Autodesk Inventor part; units mm, degrees
(part 2 of 2)
  spline S263 degree 2 poles (-39.5849, -51.31) (-39.1944, -51.6609) (-38.794, -52.3233) (-38.794, -52.7089) knots 0 0 0 1 2 2 2
  spline S264 degree 2 poles (-38.794, -52.7089) (-38.794, -53.0055) (-38.9769, -53.49) (-39.1845, -53.6679) knots 0 0 0 1 2 2 2
  spline S265 degree 2 poles (-39.1845, -53.6679) (-39.3921, -53.8508) (-40.015, -54.0535) (-40.4846, -54.0535) knots 0 0 0 1 2 2 2
  line L187 (-40.4846, -54.0535) -> (-43.5, -54.0535)
  line L188 (-43.5, -54.0535) -> (-43.5, -53.2823)
  line L189 (-43.5, -60.3265) -> (-40.8504, -60.3265)
  spline S266 degree 2 poles (-40.8504, -60.3265) (-40.534, -60.3265) (-39.9952, -60.2771) (-39.8469, -60.198) knots 0 0 0 1 2 2 2
  spline S267 degree 2 poles (-39.8469, -60.198) (-39.6838, -60.1189) (-39.5256, -59.8173) (-39.5256, -59.5553) knots 0 0 0 1 2 2 2
  spline S268 degree 2 poles (-39.5256, -59.5553) (-39.5256, -59.3181) (-39.8173, -58.7743) (-40.0941, -58.4876) knots 0 0 0 1 2 2 2
  spline S269 degree 2 poles (-40.0941, -58.4876) (-40.1633, -58.4925) (-40.3561, -58.5024) (-40.4846, -58.5024) knots 0 0 0 1 2 2 2
  line L190 (-40.4846, -58.5024) -> (-43.5, -58.5024)
  line L191 (-43.5, -58.5024) -> (-43.5, -57.7313)
  line L192 (-43.5, -57.7313) -> (-40.8504, -57.7313)
  spline S270 degree 2 poles (-40.8504, -57.7313) (-40.534, -57.7313) (-39.9952, -57.6818) (-39.8469, -57.6028) knots 0 0 0 1 2 2 2
  spline S271 degree 2 poles (-39.8469, -57.6028) (-39.6838, -57.5237) (-39.5256, -57.2221) (-39.5256, -56.9601) knots 0 0 0 1 2 2 2
  spline S272 degree 2 poles (-39.5256, -56.9601) (-39.5256, -56.713) (-39.837, -56.1643) (-40.0793, -55.9072) knots 0 0 0 1 2 2 2
  line L193 (-40.0793, -55.9072) -> (-43.5, -55.9072)
  line L194 (-43.5, -55.9072) -> (-43.5, -55.1361)
  line L195 (-43.5, -55.1361) -> (-38.9225, -55.1361)
  line L196 (-38.9225, -55.1361) -> (-38.9225, -55.9072)
  line L197 (-38.9225, -55.9072) -> (-39.4267, -55.9072)
  spline S273 degree 2 poles (-39.4267, -55.9072) (-39.1252, -56.2088) (-38.794, -56.8019) (-38.794, -57.1579) knots 0 0 0 1 2 2 2
  spline S274 degree 2 poles (-38.794, -57.1579) (-38.794, -57.5632) (-39.1647, -58.191) (-39.5849, -58.3541) knots 0 0 0 1 2 2 2
  spline S275 degree 2 poles (-39.5849, -58.3541) (-39.1944, -58.7051) (-38.794, -59.3675) (-38.794, -59.7531) knots 0 0 0 1 2 2 2
  spline S276 degree 2 poles (-38.794, -59.7531) (-38.794, -60.0497) (-38.9769, -60.5341) (-39.1845, -60.7121) knots 0 0 0 1 2 2 2
  spline S277 degree 2 poles (-39.1845, -60.7121) (-39.3921, -60.895) (-40.015, -61.0976) (-40.4846, -61.0976) knots 0 0 0 1 2 2 2
  line L198 (-40.4846, -61.0976) -> (-43.5, -61.0976)
  line L199 (-43.5, -61.0976) -> (-43.5, -60.3265)
  spline S278 degree 2 poles (-53.6384, -40.6671) (-53.6384, -40.2123) (-53.3665, -39.4659) (-53.1144, -39.2039) knots 0 0 0 1 2 2 2
  spline S279 degree 2 poles (-53.1144, -39.2039) (-52.8673, -38.9468) (-52.195, -38.6799) (-51.8143, -38.6799) knots 0 0 0 1 2 2 2
  spline S280 degree 2 poles (-51.8143, -38.6799) (-51.32, -38.6799) (-50.4895, -39.2088) (-50.2424, -39.713) knots 0 0 0 1 2 2 2
  line L200 (-50.2424, -39.713) -> (-50.2177, -39.713)
  spline S281 degree 2 poles (-50.2177, -39.713) (-49.9557, -39.2632) (-49.3328, -38.8282) (-48.8682, -38.8282) knots 0 0 0 1 2 2 2
  spline S282 degree 2 poles (-48.8682, -38.8282) (-48.181, -38.8282) (-47.2616, -39.8663) (-47.2616, -40.6671) knots 0 0 0 1 2 2 2
  spline S283 degree 2 poles (-47.2616, -40.6671) (-47.2616, -41.4976) (-48.1316, -42.5011) (-48.8138, -42.5011) knots 0 0 0 1 2 2 2
  spline S284 degree 2 poles (-48.8138, -42.5011) (-49.2241, -42.5011) (-50.0249, -42.0216) (-50.2523, -41.5717) knots 0 0 0 1 2 2 2
  line L201 (-50.2523, -41.5717) -> (-50.277, -41.5717)
  spline S285 degree 2 poles (-50.277, -41.5717) (-50.5241, -42.1056) (-51.236, -42.6543) (-51.7995, -42.6543) knots 0 0 0 1 2 2 2
  spline S286 degree 2 poles (-51.7995, -42.6543) (-52.5806, -42.6543) (-53.6384, -41.5173) (-53.6384, -40.6671) knots 0 0 0 1 2 2 2
  spline S287 degree 2 poles (-51.8786, -41.8139) (-51.5029, -41.8139) (-51.058, -41.5173) (-50.8306, -41.0972) knots 0 0 0 1 2 2 2
  spline S288 degree 2 poles (-50.8306, -41.0972) (-50.7515, -40.9588) (-50.5686, -40.4941) (-50.45, -40.2024) knots 0 0 0 1 2 2 2
  spline S289 degree 2 poles (-50.45, -40.2024) (-50.6724, -39.8663) (-51.3348, -39.5054) (-51.755, -39.5054) knots 0 0 0 1 2 2 2
  spline S290 degree 2 poles (-51.755, -39.5054) (-52.3087, -39.5054) (-53.0304, -40.1728) (-53.0304, -40.677) knots 0 0 0 1 2 2 2
  spline S291 degree 2 poles (-53.0304, -40.677) (-53.0304, -41.1911) (-52.4125, -41.8139) (-51.8786, -41.8139) knots 0 0 0 1 2 2 2
  spline S292 degree 2 poles (-48.8237, -41.7002) (-48.4134, -41.7002) (-47.8647, -41.1515) (-47.8647, -40.6622) knots 0 0 0 1 2 2 2
  spline S293 degree 2 poles (-47.8647, -40.6622) (-47.8647, -40.2173) (-48.3541, -39.6488) (-48.7742, -39.6488) knots 0 0 0 1 2 2 2
  spline S294 degree 2 poles (-48.7742, -39.6488) (-49.0758, -39.6488) (-49.4959, -39.9404) (-49.664, -40.2321) knots 0 0 0 1 2 2 2
  spline S295 degree 2 poles (-49.664, -40.2321) (-49.7332, -40.3557) (-49.9754, -40.8797) (-50.0447, -41.0922) knots 0 0 0 1 2 2 2
  spline S296 degree 2 poles (-50.0447, -41.0922) (-49.7728, -41.4481) (-49.1944, -41.7002) (-48.8237, -41.7002) knots 0 0 0 1 2 2 2
  spline S297 degree 2 poles (-50.45, -47.1972) (-52.0912, -47.1972) (-53.6285, -46.2431) (-53.6285, -45.2495) knots 0 0 0 1 2 2 2
  spline S298 degree 2 poles (-53.6285, -45.2495) (-53.6285, -44.2411) (-52.0615, -43.2969) (-50.4549, -43.2969) knots 0 0 0 1 2 2 2
  spline S299 degree 2 poles (-50.4549, -43.2969) (-48.8039, -43.2969) (-47.2764, -44.251) (-47.2764, -45.2495) knots 0 0 0 1 2 2 2
  spline S300 degree 2 poles (-47.2764, -45.2495) (-47.2764, -46.253) (-48.8583, -47.1972) (-50.45, -47.1972) knots 0 0 0 1 2 2 2
  spline S301 degree 2 poles (-52.3087, -46.1492) (-52.0071, -46.2678) (-51.0778, -46.3667) (-50.45, -46.3667) knots 0 0 0 1 2 2 2
  spline S302 degree 2 poles (-50.45, -46.3667) (-49.8222, -46.3667) (-48.8978, -46.2678) (-48.5864, -46.1442) knots 0 0 0 1 2 2 2
  spline S303 degree 2 poles (-48.5864, -46.1442) (-48.275, -46.0207) (-47.9536, -45.5906) (-47.9536, -45.2495) knots 0 0 0 1 2 2 2
  spline S304 degree 2 poles (-47.9536, -45.2495) (-47.9536, -44.9084) (-48.275, -44.4685) (-48.5963, -44.34) knots 0 0 0 1 2 2 2
  spline S305 degree 2 poles (-48.5963, -44.34) (-48.9077, -44.2164) (-49.8568, -44.1274) (-50.4549, -44.1274) knots 0 0 0 1 2 2 2
  spline S306 degree 2 poles (-50.4549, -44.1274) (-51.0976, -44.1274) (-51.9577, -44.2065) (-52.2938, -44.335) knots 0 0 0 1 2 2 2
  spline S307 degree 2 poles (-52.2938, -44.335) (-52.6102, -44.4536) (-52.9513, -44.8936) (-52.9513, -45.2495) knots 0 0 0 1 2 2 2
  spline S308 degree 2 poles (-52.9513, -45.2495) (-52.9513, -45.5857) (-52.63, -46.0256) (-52.3087, -46.1492) knots 0 0 0 1 2 2 2
  line L202 (-53.5, -53.2823) -> (-50.8504, -53.2823)
  spline S309 degree 2 poles (-50.8504, -53.2823) (-50.534, -53.2823) (-49.9952, -53.2329) (-49.8469, -53.1538) knots 0 0 0 1 2 2 2
  spline S310 degree 2 poles (-49.8469, -53.1538) (-49.6838, -53.0747) (-49.5256, -52.7732) (-49.5256, -52.5112) knots 0 0 0 1 2 2 2
  spline S311 degree 2 poles (-49.5256, -52.5112) (-49.5256, -52.2739) (-49.8173, -51.7301) (-50.0941, -51.4434) knots 0 0 0 1 2 2 2
  spline S312 degree 2 poles (-50.0941, -51.4434) (-50.1633, -51.4484) (-50.3561, -51.4583) (-50.4846, -51.4583) knots 0 0 0 1 2 2 2
  line L203 (-50.4846, -51.4583) -> (-53.5, -51.4583)
  line L204 (-53.5, -51.4583) -> (-53.5, -50.6871)
  line L205 (-53.5, -50.6871) -> (-50.8504, -50.6871)
  spline S313 degree 2 poles (-50.8504, -50.6871) (-50.534, -50.6871) (-49.9952, -50.6377) (-49.8469, -50.5586) knots 0 0 0 1 2 2 2
  spline S314 degree 2 poles (-49.8469, -50.5586) (-49.6838, -50.4795) (-49.5256, -50.178) (-49.5256, -49.916) knots 0 0 0 1 2 2 2
  spline S315 degree 2 poles (-49.5256, -49.916) (-49.5256, -49.6688) (-49.837, -49.1201) (-50.0793, -48.863) knots 0 0 0 1 2 2 2
  line L206 (-50.0793, -48.863) -> (-53.5, -48.863)
  line L207 (-53.5, -48.863) -> (-53.5, -48.0919)
  line L208 (-53.5, -48.0919) -> (-48.9225, -48.0919)
  line L209 (-48.9225, -48.0919) -> (-48.9225, -48.863)
  line L210 (-48.9225, -48.863) -> (-49.4267, -48.863)
  spline S316 degree 2 poles (-49.4267, -48.863) (-49.1252, -49.1646) (-48.794, -49.7578) (-48.794, -50.1137) knots 0 0 0 1 2 2 2
  spline S317 degree 2 poles (-48.794, -50.1137) (-48.794, -50.519) (-49.1647, -51.1468) (-49.5849, -51.31) knots 0 0 0 1 2 2 2
  spline S318 degree 2 poles (-49.5849, -51.31) (-49.1944, -51.6609) (-48.794, -52.3233) (-48.794, -52.7089) knots 0 0 0 1 2 2 2
  spline S319 degree 2 poles (-48.794, -52.7089) (-48.794, -53.0055) (-48.9769, -53.49) (-49.1845, -53.6679) knots 0 0 0 1 2 2 2
  spline S320 degree 2 poles (-49.1845, -53.6679) (-49.3921, -53.8508) (-50.015, -54.0535) (-50.4846, -54.0535) knots 0 0 0 1 2 2 2
  line L211 (-50.4846, -54.0535) -> (-53.5, -54.0535)
  line L212 (-53.5, -54.0535) -> (-53.5, -53.2823)
  line L213 (-53.5, -60.3265) -> (-50.8504, -60.3265)
  spline S321 degree 2 poles (-50.8504, -60.3265) (-50.534, -60.3265) (-49.9952, -60.2771) (-49.8469, -60.198) knots 0 0 0 1 2 2 2
  spline S322 degree 2 poles (-49.8469, -60.198) (-49.6838, -60.1189) (-49.5256, -59.8173) (-49.5256, -59.5553) knots 0 0 0 1 2 2 2
  spline S323 degree 2 poles (-49.5256, -59.5553) (-49.5256, -59.3181) (-49.8173, -58.7743) (-50.0941, -58.4876) knots 0 0 0 1 2 2 2
  spline S324 degree 2 poles (-50.0941, -58.4876) (-50.1633, -58.4925) (-50.3561, -58.5024) (-50.4846, -58.5024) knots 0 0 0 1 2 2 2
  line L214 (-50.4846, -58.5024) -> (-53.5, -58.5024)
  line L215 (-53.5, -58.5024) -> (-53.5, -57.7313)
  line L216 (-53.5, -57.7313) -> (-50.8504, -57.7313)
  spline S325 degree 2 poles (-50.8504, -57.7313) (-50.534, -57.7313) (-49.9952, -57.6818) (-49.8469, -57.6028) knots 0 0 0 1 2 2 2
  spline S326 degree 2 poles (-49.8469, -57.6028) (-49.6838, -57.5237) (-49.5256, -57.2221) (-49.5256, -56.9601) knots 0 0 0 1 2 2 2
  spline S327 degree 2 poles (-49.5256, -56.9601) (-49.5256, -56.713) (-49.837, -56.1643) (-50.0793, -55.9072) knots 0 0 0 1 2 2 2
  line L217 (-50.0793, -55.9072) -> (-53.5, -55.9072)
  line L218 (-53.5, -55.9072) -> (-53.5, -55.1361)
  line L219 (-53.5, -55.1361) -> (-48.9225, -55.1361)
  line L220 (-48.9225, -55.1361) -> (-48.9225, -55.9072)
  line L221 (-48.9225, -55.9072) -> (-49.4267, -55.9072)
  spline S328 degree 2 poles (-49.4267, -55.9072) (-49.1252, -56.2088) (-48.794, -56.8019) (-48.794, -57.1579) knots 0 0 0 1 2 2 2
  spline S329 degree 2 poles (-48.794, -57.1579) (-48.794, -57.5632) (-49.1647, -58.191) (-49.5849, -58.3541) knots 0 0 0 1 2 2 2
  spline S330 degree 2 poles (-49.5849, -58.3541) (-49.1944, -58.7051) (-48.794, -59.3675) (-48.794, -59.7531) knots 0 0 0 1 2 2 2
  spline S331 degree 2 poles (-48.794, -59.7531) (-48.794, -60.0497) (-48.9769, -60.5341) (-49.1845, -60.7121) knots 0 0 0 1 2 2 2
  spline S332 degree 2 poles (-49.1845, -60.7121) (-49.3921, -60.895) (-50.015, -61.0976) (-50.4846, -61.0976) knots 0 0 0 1 2 2 2
  line L222 (-50.4846, -61.0976) -> (-53.5, -61.0976)
  line L223 (-53.5, -61.0976) -> (-53.5, -60.3265)
  spline S333 degree 2 poles (-59.3823, -38.6552) (-58.9126, -38.6552) (-58.1316, -38.9617) (-57.8498, -39.2286) knots 0 0 0 1 2 2 2
  spline S334 degree 2 poles (-57.8498, -39.2286) (-57.578, -39.4807) (-57.2764, -40.2173) (-57.2764, -40.5929) knots 0 0 0 1 2 2 2
  spline S335 degree 2 poles (-57.2764, -40.5929) (-57.2764, -41.0131) (-57.5582, -41.6953) (-57.8251, -41.9474) knots 0 0 0 1 2 2 2
  spline S336 degree 2 poles (-57.8251, -41.9474) (-58.1613, -42.2638) (-59.2488, -42.6098) (-60.0842, -42.6098) knots 0 0 0 1 2 2 2
  spline S337 degree 2 poles (-60.0842, -42.6098) (-60.8405, -42.6098) (-62.195, -42.2687) (-62.6448, -41.9375) knots 0 0 0 1 2 2 2
  spline S338 degree 2 poles (-62.6448, -41.9375) (-63.1194, -41.5865) (-63.6186, -40.5979) (-63.6186, -39.8762) knots 0 0 0 1 2 2 2
  spline S339 degree 2 poles (-63.6186, -39.8762) (-63.6186, -39.713) (-63.584, -39.3423) (-63.5346, -39.1841) knots 0 0 0 1 2 2 2
  line L224 (-63.5346, -39.1841) -> (-62.7486, -39.1841)
  line L225 (-62.7486, -39.1841) -> (-62.7486, -39.2237)
  spline S340 degree 2 poles (-62.7486, -39.2237) (-62.8079, -39.3275) (-62.9118, -39.7625) (-62.9118, -39.9849) knots 0 0 0 1 2 2 2
  spline S341 degree 2 poles (-62.9118, -39.9849) (-62.9118, -40.7857) (-61.8539, -41.7002) (-60.8751, -41.7645) knots 0 0 0 1 2 2 2
  spline S342 degree 2 poles (-60.8751, -41.7645) (-61.0976, -41.4382) (-61.3002, -40.8451) (-61.3002, -40.4941) knots 0 0 0 1 2 2 2
  spline S343 degree 2 poles (-61.3002, -40.4941) (-61.3002, -40.1579) (-61.1519, -39.5994) (-60.9394, -39.3176) knots 0 0 0 1 2 2 2
  spline S344 degree 2 poles (-60.9394, -39.3176) (-60.6873, -38.9913) (-59.9211, -38.6552) (-59.3823, -38.6552) knots 0 0 0 1 2 2 2
  spline S345 degree 2 poles (-59.9013, -41.7843) (-59.2834, -41.7843) (-58.5023, -41.5569) (-58.2898, -41.3542) knots 0 0 0 1 2 2 2
  spline S346 degree 2 poles (-58.2898, -41.3542) (-58.0921, -41.1763) (-57.9438, -40.8055) (-57.9438, -40.588) knots 0 0 0 1 2 2 2
  spline S347 degree 2 poles (-57.9438, -40.588) (-57.9438, -40.0838) (-58.6655, -39.4857) (-59.3476, -39.4857) knots 0 0 0 1 2 2 2
  spline S348 degree 2 poles (-59.3476, -39.4857) (-59.7332, -39.4857) (-60.2325, -39.6834) (-60.4105, -39.9009) knots 0 0 0 1 2 2 2
  spline S349 degree 2 poles (-60.4105, -39.9009) (-60.539, -40.0591) (-60.623, -40.4496) (-60.623, -40.677) knots 0 0 0 1 2 2 2
  spline S350 degree 2 poles (-60.623, -40.677) (-60.623, -40.939) (-60.4401, -41.5421) (-60.2869, -41.7694) knots 0 0 0 1 2 2 2
  spline S351 degree 2 poles (-60.2869, -41.7694) (-60.2276, -41.7744) (-60.0249, -41.7843) (-59.9013, -41.7843) knots 0 0 0 1 2 2 2
  spline S352 degree 2 poles (-60.45, -47.1972) (-62.0912, -47.1972) (-63.6285, -46.2431) (-63.6285, -45.2495) knots 0 0 0 1 2 2 2
  spline S353 degree 2 poles (-63.6285, -45.2495) (-63.6285, -44.2411) (-62.0615, -43.2969) (-60.4549, -43.2969) knots 0 0 0 1 2 2 2
  spline S354 degree 2 poles (-60.4549, -43.2969) (-58.8039, -43.2969) (-57.2764, -44.251) (-57.2764, -45.2495) knots 0 0 0 1 2 2 2
  spline S355 degree 2 poles (-57.2764, -45.2495) (-57.2764, -46.253) (-58.8583, -47.1972) (-60.45, -47.1972) knots 0 0 0 1 2 2 2
  spline S356 degree 2 poles (-62.3087, -46.1492) (-62.0071, -46.2678) (-61.0778, -46.3667) (-60.45, -46.3667) knots 0 0 0 1 2 2 2
  spline S357 degree 2 poles (-60.45, -46.3667) (-59.8222, -46.3667) (-58.8978, -46.2678) (-58.5864, -46.1442) knots 0 0 0 1 2 2 2
  spline S358 degree 2 poles (-58.5864, -46.1442) (-58.275, -46.0207) (-57.9536, -45.5906) (-57.9536, -45.2495) knots 0 0 0 1 2 2 2
  spline S359 degree 2 poles (-57.9536, -45.2495) (-57.9536, -44.9084) (-58.275, -44.4685) (-58.5963, -44.34) knots 0 0 0 1 2 2 2
  spline S360 degree 2 poles (-58.5963, -44.34) (-58.9077, -44.2164) (-59.8568, -44.1274) (-60.4549, -44.1274) knots 0 0 0 1 2 2 2
  spline S361 degree 2 poles (-60.4549, -44.1274) (-61.0976, -44.1274) (-61.9577, -44.2065) (-62.2938, -44.335) knots 0 0 0 1 2 2 2
  spline S362 degree 2 poles (-62.2938, -44.335) (-62.6102, -44.4536) (-62.9513, -44.8936) (-62.9513, -45.2495) knots 0 0 0 1 2 2 2
  spline S363 degree 2 poles (-62.9513, -45.2495) (-62.9513, -45.5857) (-62.63, -46.0256) (-62.3087, -46.1492) knots 0 0 0 1 2 2 2
  line L226 (-63.5, -53.2823) -> (-60.8504, -53.2823)
  spline S364 degree 2 poles (-60.8504, -53.2823) (-60.534, -53.2823) (-59.9952, -53.2329) (-59.8469, -53.1538) knots 0 0 0 1 2 2 2
  spline S365 degree 2 poles (-59.8469, -53.1538) (-59.6838, -53.0747) (-59.5256, -52.7732) (-59.5256, -52.5112) knots 0 0 0 1 2 2 2
  spline S366 degree 2 poles (-59.5256, -52.5112) (-59.5256, -52.2739) (-59.8173, -51.7301) (-60.0941, -51.4434) knots 0 0 0 1 2 2 2
  spline S367 degree 2 poles (-60.0941, -51.4434) (-60.1633, -51.4484) (-60.3561, -51.4583) (-60.4846, -51.4583) knots 0 0 0 1 2 2 2
  line L227 (-60.4846, -51.4583) -> (-63.5, -51.4583)
  line L228 (-63.5, -51.4583) -> (-63.5, -50.6871)
  line L229 (-63.5, -50.6871) -> (-60.8504, -50.6871)
  spline S368 degree 2 poles (-60.8504, -50.6871) (-60.534, -50.6871) (-59.9952, -50.6377) (-59.8469, -50.5586) knots 0 0 0 1 2 2 2
  spline S369 degree 2 poles (-59.8469, -50.5586) (-59.6838, -50.4795) (-59.5256, -50.178) (-59.5256, -49.916) knots 0 0 0 1 2 2 2
  spline S370 degree 2 poles (-59.5256, -49.916) (-59.5256, -49.6688) (-59.837, -49.1201) (-60.0793, -48.863) knots 0 0 0 1 2 2 2
  line L230 (-60.0793, -48.863) -> (-63.5, -48.863)
  line L231 (-63.5, -48.863) -> (-63.5, -48.0919)
  line L232 (-63.5, -48.0919) -> (-58.9225, -48.0919)
  line L233 (-58.9225, -48.0919) -> (-58.9225, -48.863)
  line L234 (-58.9225, -48.863) -> (-59.4267, -48.863)
  spline S371 degree 2 poles (-59.4267, -48.863) (-59.1252, -49.1646) (-58.794, -49.7578) (-58.794, -50.1137) knots 0 0 0 1 2 2 2
  spline S372 degree 2 poles (-58.794, -50.1137) (-58.794, -50.519) (-59.1647, -51.1468) (-59.5849, -51.31) knots 0 0 0 1 2 2 2
  spline S373 degree 2 poles (-59.5849, -51.31) (-59.1944, -51.6609) (-58.794, -52.3233) (-58.794, -52.7089) knots 0 0 0 1 2 2 2
  spline S374 degree 2 poles (-58.794, -52.7089) (-58.794, -53.0055) (-58.9769, -53.49) (-59.1845, -53.6679) knots 0 0 0 1 2 2 2
  spline S375 degree 2 poles (-59.1845, -53.6679) (-59.3921, -53.8508) (-60.015, -54.0535) (-60.4846, -54.0535) knots 0 0 0 1 2 2 2
  line L235 (-60.4846, -54.0535) -> (-63.5, -54.0535)
  line L236 (-63.5, -54.0535) -> (-63.5, -53.2823)
  line L237 (-63.5, -60.3265) -> (-60.8504, -60.3265)
  spline S376 degree 2 poles (-60.8504, -60.3265) (-60.534, -60.3265) (-59.9952, -60.2771) (-59.8469, -60.198) knots 0 0 0 1 2 2 2
  spline S377 degree 2 poles (-59.8469, -60.198) (-59.6838, -60.1189) (-59.5256, -59.8173) (-59.5256, -59.5553) knots 0 0 0 1 2 2 2
  spline S378 degree 2 poles (-59.5256, -59.5553) (-59.5256, -59.3181) (-59.8173, -58.7743) (-60.0941, -58.4876) knots 0 0 0 1 2 2 2
  spline S379 degree 2 poles (-60.0941, -58.4876) (-60.1633, -58.4925) (-60.3561, -58.5024) (-60.4846, -58.5024) knots 0 0 0 1 2 2 2
  line L238 (-60.4846, -58.5024) -> (-63.5, -58.5024)
  line L239 (-63.5, -58.5024) -> (-63.5, -57.7313)
  line L240 (-63.5, -57.7313) -> (-60.8504, -57.7313)
  spline S380 degree 2 poles (-60.8504, -57.7313) (-60.534, -57.7313) (-59.9952, -57.6818) (-59.8469, -57.6028) knots 0 0 0 1 2 2 2
  spline S381 degree 2 poles (-59.8469, -57.6028) (-59.6838, -57.5237) (-59.5256, -57.2221) (-59.5256, -56.9601) knots 0 0 0 1 2 2 2
  spline S382 degree 2 poles (-59.5256, -56.9601) (-59.5256, -56.713) (-59.837, -56.1643) (-60.0793, -55.9072) knots 0 0 0 1 2 2 2
  line L241 (-60.0793, -55.9072) -> (-63.5, -55.9072)
  line L242 (-63.5, -55.9072) -> (-63.5, -55.1361)
  line L243 (-63.5, -55.1361) -> (-58.9225, -55.1361)
  line L244 (-58.9225, -55.1361) -> (-58.9225, -55.9072)
  line L245 (-58.9225, -55.9072) -> (-59.4267, -55.9072)
  spline S383 degree 2 poles (-59.4267, -55.9072) (-59.1252, -56.2088) (-58.794, -56.8019) (-58.794, -57.1579) knots 0 0 0 1 2 2 2
  spline S384 degree 2 poles (-58.794, -57.1579) (-58.794, -57.5632) (-59.1647, -58.191) (-59.5849, -58.3541) knots 0 0 0 1 2 2 2
  spline S385 degree 2 poles (-59.5849, -58.3541) (-59.1944, -58.7051) (-58.794, -59.3675) (-58.794, -59.7531) knots 0 0 0 1 2 2 2
  spline S386 degree 2 poles (-58.794, -59.7531) (-58.794, -60.0497) (-58.9769, -60.5341) (-59.1845, -60.7121) knots 0 0 0 1 2 2 2
  spline S387 degree 2 poles (-59.1845, -60.7121) (-59.3921, -60.895) (-60.015, -61.0976) (-60.4846, -61.0976) knots 0 0 0 1 2 2 2
  line L246 (-60.4846, -61.0976) -> (-63.5, -61.0976)
  line L247 (-63.5, -61.0976) -> (-63.5, -60.3265)
  point P0 (0, 0)
  dimension "d20" = 20
  constraints: 16 end point, 13 vertical, 3 parallel
  measures "d20" distance from line of A3.centre L2
emboss "Emboss1" sketch "Sketch4" operation cut depth 1 direction (0, 0, -1)
equation "\"d11\" = d10"
equation "\"d12\" = d10"
equation "\"d13\" = d10"
equation "\"d14\" = d10"
body "Solid1"
